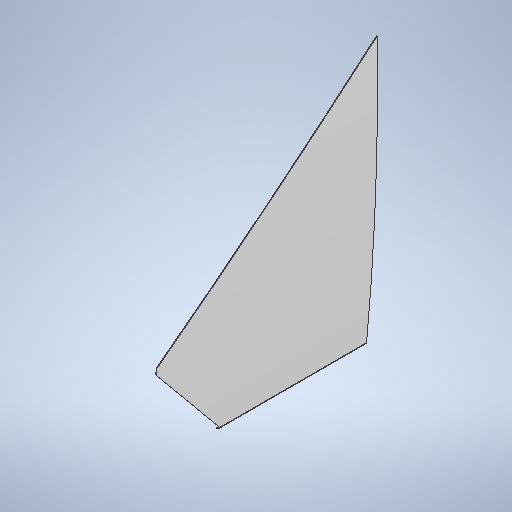
# Autodesk Inventor part: MSC 027 sheet left-right board face 1
Saved by Autodesk Inventor 2025 (Build 290162010, 162A)
## iProperties
Created: 2024-04-18
Part Number: MSC 027 sheet left-right board face 1
Material: AISI304
Document SubType Name: Sheet Metal
Designer: admin
Stock Number: МОО 027 лист левый-правый борт морда 1
Mass: 48027.3 g
Surface Area: 40202.8 cm^2
Volume: 6003.41 cm^3
Density: 8 g/cm^3
Sheet Metal Rule: Default_mm
Sheet Metal Width: 0,000 mm
Sheet Metal Length: 0,000 mm
Sheet Metal Area: 0,000 mm^2
Appearance: Default
Author: admin
Autodesk Inventor part; units mm, degrees
ref_plane "YZ Plane" through (0, 0, 0) normal (1, 0, 0) x (0, 1, 0)
ref_plane "XZ Plane" through (0, 0, 0) normal (0, 1, 0) x (-1, 0, 0)
ref_plane "XY Plane" through (0, 0, 0) normal (0, 0, 1) x (1, 0, 0)
sketch "Sketch1" plane through (0, 0, 0) normal (0, 0, 1) x (1, 0, 0)
  line L0 (-750, 0) -> (750, 0) construction
  line L1 (750, 0) -> (750, -2700) construction
  line L2 (750, -2700) -> (-750, -2700) construction
  line L3 (-750, -2700) -> (-750, 0) construction
  line L4 (800, 50) -> (-800, 50) construction
  line L5 (-800, 50) -> (-800, -2750) construction
  line L6 (-800, -2750) -> (800, -2750) construction
  line L7 (800, -2750) -> (800, 50) construction
  line L8 (-850, 100) -> (850, 100) construction
  line L9 (850, 100) -> (850, -2800) construction
  line L10 (850, -2800) -> (-850, -2800) construction
  line L11 (-850, -2800) -> (-850, 100) construction
  line L12 (-750, -2100) -> (750, -2100) construction
  line L13 (115.485997, -2697.8227) -> (682.456682, -2163.637569) construction
  arc A0 (750, -2100) -> (750.178737, -2098.125829) centre (-10250, -1050) ccw construction
  arc A1 (748.630029, -2101.290751) -> (750.178737, -2098.125829) centre (745.201281, -2097.651564) ccw
  arc A2 (110, -2700) -> (115.485997, -2697.8227) centre (110, -2692) ccw construction
  line L14 (15976.068527, -18395.893169) -> (682.456682, -2163.637569) construction
  arc A3 (750, 0) -> (0, 50) centre (0, -5600) ccw construction
  line L15 (0, 100) -> (0, 50) construction
  line L16 (0, -2700) -> (0, -12420.16254) construction
  line L17 (0, -9674.941914) -> (0, 0) construction
  line L18 (682.456682, -2163.637569) -> (748.630029, -2101.290751)
  arc A4 (750.178737, -2098.125829) -> (768.550013, -216.9) centre (-10250, -1050) ccw
  line L19 (748.630029, -2101.290751) -> (750, -2100) construction
  line L20 (768.550013, -216.9) -> (750, 0) construction
  point P0 (0, -2750)
  dimension "d129" = 1500
  dimension "d130" = 2700
  dimension "d131" = 2100
  dimension "d132" = 5
  dimension "d133" = 8
  dimension "d134" = 50
  dimension "d135" = 50
  dimension "d136" = 110
  dimension "d137" = 92.8
  dimension "d138" = 216.9
  measures "d129" distance of L3.end L20.end
  measures "d130" distance of L20.end L1.end
  measures "d131" distance between parallel lines of L12 L0
  measures "d132" radius of A1
  measures "d133" radius of A2
  measures "d134" distance between parallel lines of L4 L8
  measures "d135" distance between parallel lines of L0 L4
  measures "d136" distance from line of L16 A2.centre
  measures "d137" distance of L12.end L18.start
  measures "d138" vertical distance of L20.start L20.end
contour flange "Contour Flange2" sketch "Sketch1" thickness 3 bend radius 3 width 980 along (0, 0, 1) mid plane no both sides no wall seen from (715.543355, -2132.46416, 0) lies toward (0.6857497, -0.7278375, 0) curves L18 A1 A4
bend "Bend2"
corner "Corner2"
sketch "Sketch2" plane through (0, 0, 0) normal (1, 0, 0) x (0, 1, 0)
  line L0 (-2098.410388, 980) -> (-2098.410388, 0)
  line L1 (-2098.410388, 0) -> (-216.673819, 0)
  line L2 (-216.673819, 0) -> (-216.673819, 980)
  line L3 (-2098.410388, 980) -> (-216.673819, 980)
  line L4 (-2103.474264, 980) -> (-2103.474264, 0)
  line L5 (-2165.821082, 980) -> (-2103.474264, 980)
  line L6 (-2165.821082, 0) -> (-2165.821082, 980)
  line L7 (-2165.821082, 0) -> (-2103.474264, 0)
  line L8 (-2098.410388, 0) -> (-2103.474264, 0)
  line L9 (-2098.410388, 980) -> (-2103.474264, 980)
  line L10 (-872.673819, 980) -> (-1694.991458, 0)
  line L11 (-872.673819, 0) -> (-1694.991458, 980)
  line L12 (-1722.439791, 980) -> (-2165.821082, 607.958923)
  line L13 (-1722.439791, 0) -> (-2165.821082, 372.041077)
  point P0 (0, 0)
  point P1 (-1283.832638, 490)
  dimension "d150" = 40
  dimension "d151" = 285
  dimension "d152" = 656
  constraints: 12 end point, 8 point on line, 2 equal length, 2 midpoint, 2 perpendicular, 1 horizontal
  measures "d150" angle of L3 L12
  measures "d151" distance from line of L12 L5.start
  measures "d152" distance of L11.start L1.end
extrude "Extrusion2" cut sketch "Sketch2" along normal through all both and the other way through all contours L3 L12 L0 | L0 L12 L4 L9 | L4 L12 L6 L5 | L3 L10 L11 | L3 L2 L1 L11 L10
sketch "Sketch4" plane through (749.1768, -2100.77463, 662.50511) normal (-0.6852958, 0.7282648, 0) x (0.7282648, 0.6852958, 0)
  line L0 (-59.382943, 165.716241) -> (-59.382943, 507.035792) construction
  line L1 (-59.382943, 507.035792) -> (-32.420537, 507.035792) construction
  line L2 (-32.420537, 507.035792) -> (-32.420537, 165.716241) construction
  line L3 (-32.420537, 165.716241) -> (-59.382943, 165.716241) construction
  point P0 (894.052911, 662.50511)
  constraints: 2 other
mark "Mark2"
equation "\"d36\" = Thickness"
equation "\"d37\" = BendReliefWidth"
equation "\"d38\" = BendReliefDepth"
equation "\"d39\" = MinimumRemnant"
equation "\"d40\" = TransitionRadius"
equation "\"d42\" = BendRadius"
equation "\"d44\" = CornerReliefSize"
equation "\"d45\" = GapSize"
equation "\"d46\" = JacobiRadiusSize"
equation "\"BendRadius\" = Thickness"
equation "\"BendReliefWidth\" = Thickness"
equation "\"BendReliefDepth\" = 0.5 * Thickness"
equation "\"CornerReliefSize\" = 4 * Thickness"
equation "\"MinimumRemnant\" = 2 * Thickness"
equation "\"TransitionRadius\" = BendRadius"
equation "\"JacobiRadiusSize\" = BendRadius"
equation "\"GapSize\" = Thickness"
equation "\"Thickness\" = 3"
body "Solid3"
